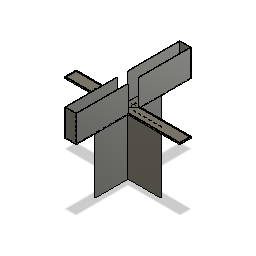
EPM (Autodesk Fusion 360 design; units mm, degrees)
Autodesk Fusion 360 part; units mm, degrees
note: some values were not read from the file. Chosen so that the rebuilt part matches the saved one: which bodies a step acts on. Set by a fixed rule: which sketch regions a step uses.
sketch "Maze" plane through (0, 0, 0) normal (0, 1, 0) x (1, 0, 0) in component "Main"
  line L0 (-50, 50) -> (50, 50) construction
  line L1 (50, 50) -> (50, -50) construction
  line L2 (50, -50) -> (-50, -50)
  line L3 (-50, -50) -> (-50, 50) construction
  line L4 (-50, 50) -> (-50, 550)
  line L5 (-50, 550) -> (50, 550)
  line L6 (50, 550) -> (50, 50)
  line L7 (50, 50) -> (550, 50)
  line L8 (550, 50) -> (550, -50)
  line L9 (550, -50) -> (50, -50)
  line L10 (-50, 50) -> (50, -50)
  line L11 (55.8, 55.8) -> (555.8, 55.8)
  line L12 (555.8, 55.8) -> (555.8, -55.8)
  line L13 (555.8, -55.8) -> (55.8, -55.8)
  line L14 (-50, -50) -> (-50, -550)
  line L15 (-50, -550) -> (50, -550)
  line L16 (50, -550) -> (50, -50)
  line L17 (55.8, -55.8) -> (55.8, -555.8)
  line L18 (55.8, -555.8) -> (-55.8, -555.8)
  line L19 (-50, 50) -> (-550, 50)
  line L20 (-550, 50) -> (-550, -50)
  line L21 (-550, -50) -> (-50, -50)
  line L22 (55.8, 55.8) -> (55.8, 555.8)
  line L23 (55.8, 555.8) -> (-55.8, 555.8)
  line L24 (-55.8, 555.8) -> (-55.8, 55.8)
  line L25 (-55.8, 55.8) -> (-555.8, 55.8)
  line L26 (-555.8, 55.8) -> (-555.8, -55.8)
  line L27 (-555.8, -55.8) -> (-55.8, -55.8)
  line L28 (-55.8, -55.8) -> (-55.8, -555.8)
  line L29 (-55.8, 55.8) -> (-50, 55.8)
  line L30 (-55.8, 55.8) -> (-55.8, 50)
  line L31 (55.8, 55.8) -> (50, 55.8)
  line L32 (55.8, 55.8) -> (55.8, 50)
  line L33 (-55.8, -55.8) -> (-55.8, -50)
  line L34 (-55.8, -55.8) -> (-50, -55.8)
  line L35 (55.8, -55.8) -> (55.8, -50)
  line L36 (55.8, -55.8) -> (50, -55.8)
  line L37 (-50, 550) -> (-50, 555.8)
  line L38 (550, 50) -> (555.8, 50)
  line L39 (50, -550) -> (50, -555.8)
  line L40 (-550, -50) -> (-555.8, -50)
  line L41 (-50, -50) -> (50, 50)
  line L42 (550, 50) -> (550, 55.8)
  line L43 (550, -50) -> (555.8, -50)
  line L44 (555.8, -50) -> (550, -50)
  line L45 (550, -50) -> (550, -55.8)
  line L46 (50, -550) -> (55.8, -550)
  line L47 (-50, -550) -> (-50, -555.8)
  line L48 (-50, -550) -> (-55.8, -550)
  line L49 (-550, -50) -> (-550, -55.8)
  line L50 (-550, 50) -> (-550, 55.8)
  line L51 (-550, 55.8) -> (-550, 50)
  line L52 (-555.8, 50) -> (-550, 50)
  line L53 (-50, 550) -> (-55.8, 550)
  line L54 (50, 550) -> (55.8, 550)
  line L55 (50, 550) -> (50, 555.8)
  line L56 (-55.8, 75.8) -> (-50, 75.8)
  line L57 (50, 75.8) -> (55.8, 75.8)
  line L58 (75.8, 55.8) -> (75.8, 50)
  line L59 (75.8, -50) -> (75.8, -55.8)
  line L60 (-50, 75.8) -> (50, 75.8) construction
  line L61 (75.8, 50) -> (75.8, -50) construction
  line L62 (-52.9, 75.8) -> (-52.9, 55.8) construction
  line L63 (75.8, 52.9) -> (55.8, 52.9) construction
  line L64 (-30, 555.8) -> (-30, 550)
  line L65 (-30, 552.9) -> (-50, 552.9) construction
  line L66 (550, 30) -> (555.8, 30)
  line L67 (552.9, 30) -> (552.9, 50) construction
  line L68 (2.9, 2.9) -> (-2.9, 2.9)
  line L69 (-2.9, 2.9) -> (-2.9, -2.9)
  line L70 (-2.9, -2.9) -> (2.9, -2.9)
  line L71 (2.9, -2.9) -> (2.9, 2.9)
  dimension "d8" = 100
  dimension "d9" = 500
  dimension "d13" = 5.8
  dimension "d33" = 20
  dimension "d34" = 20
  dimension "d108" = 5.8
  constraint horizontal L0
  constraint vertical L1
  constraint horizontal L2
  constraint vertical L3
  constraint perpendicular L0 L4
  constraint perpendicular L4 L5
  constraint perpendicular L0 L6
  constraint perpendicular L1 L7
  constraint perpendicular L7 L8
  constraint perpendicular L1 L9
  constraint equal L2 L3
  constraint midpoint origin L10
  constraint parallel L7 L11
  constraint perpendicular L11 L12
  constraint perpendicular L12 L13
  constraint perpendicular L2 L14
  constraint perpendicular L14 L15
  constraint perpendicular L13 L16
  constraint perpendicular L13 L17
  constraint perpendicular L17 L18
  constraint perpendicular L4 L19
  constraint perpendicular L19 L20
  constraint perpendicular L14 L21
  constraint equal L4 L19
  constraint equal L9 L19
  constraint equal L9 L16
  constraint perpendicular L11 L22
  constraint perpendicular L6 L23
  constraint perpendicular L23 L24
  constraint perpendicular L24 L25
  constraint perpendicular L25 L26
  constraint perpendicular L24 L27
  constraint perpendicular L15 L28
  constraint coincident L4 L29.end
  constraint perpendicular L4 L29
  constraint coincident L19 L30.end
  constraint perpendicular L19 L30
  constraint coincident L6 L31.end
  constraint perpendicular L6 L31
  constraint coincident L7 L32.end
  constraint perpendicular L7 L32
  constraint coincident L21 L33.end
  constraint perpendicular L21 L33
  constraint coincident L14 L34.end
  constraint perpendicular L14 L34
  constraint coincident L9 L35.end
  constraint perpendicular L9 L35
  constraint coincident L16 L36.end
  constraint perpendicular L16 L36
  constraint coincident L23 L37.end
  constraint perpendicular L23 L37
  constraint coincident L12 L38.end
  constraint perpendicular L12 L38
  constraint coincident L18 L39.end
  constraint perpendicular L18 L39
  constraint coincident L26 L40.end
  constraint perpendicular L26 L40
  constraint equal L29 L30
  constraint equal L29 L31
  constraint equal L31 L32
  constraint equal L32 L35
  constraint equal L35 L36
  constraint equal L34 L36
  constraint equal L33 L34
  constraint equal L33 L37
  constraint equal L37 L38
  constraint equal L38 L39
  constraint equal L39 L40
  constraint coincident L11 L42.end
  constraint perpendicular L11 L42
  constraint coincident L12 L43.end
  constraint perpendicular L12 L43
  constraint coincident L13 L45.end
  constraint perpendicular L13 L45
  constraint coincident L17 L46.end
  constraint perpendicular L17 L46
  constraint coincident L18 L47.end
  constraint perpendicular L18 L47
  constraint coincident L28 L48.end
  constraint perpendicular L28 L48
  constraint coincident L27 L49.end
  constraint perpendicular L27 L49
  constraint coincident L25 L50.end
  constraint perpendicular L25 L50
  constraint coincident L26 L52.start
  constraint perpendicular L50 L52
  constraint coincident L24 L53.end
  constraint perpendicular L24 L53
  constraint coincident L22 L54.end
  constraint perpendicular L22 L54
  constraint coincident L23 L55.end
  constraint perpendicular L23 L55
  constraint coincident L24 L56.start
  constraint coincident L4 L56.end
  constraint perpendicular L4 L56
  constraint coincident L6 L57.start
  constraint coincident L22 L57.end
  constraint perpendicular L22 L57
  constraint coincident L11 L58.start
  constraint coincident L7 L58.end
  constraint perpendicular L7 L58
  constraint coincident L9 L59.start
  constraint coincident L13 L59.end
  constraint perpendicular L13 L59
  constraint perpendicular L6 L60
  constraint perpendicular L7 L61
  constraint midpoint L56 L62.start
  constraint midpoint L29 L62.end
  constraint midpoint L58 L63.start
  constraint midpoint L32 L63.end
  constraint equal L62 L63
  constraint coincident L23 L64.start
  constraint coincident L5 L64.end
  constraint perpendicular L5 L64
  constraint midpoint L64 L65.start
  constraint midpoint L37 L65.end
  constraint coincident L8 L66.start
  constraint coincident L12 L66.end
  constraint perpendicular L12 L66
  constraint midpoint L66 L67.start
  constraint midpoint L38 L67.end
  constraint equal L65 L67
  constraint horizontal L68
  constraint vertical L69
  constraint horizontal L70
  constraint vertical L71
  constraint coincident L41 L69.end
  constraint coincident L41 L68.start
  constraint coincident L10 L68.end
  measures "d8" distance of L4.end L5.end
  measures "d9" distance of L0.start L4.end
  measures "d13" distance of L4.end L37.end
  measures "d33" distance of L62.start L62.end
  measures "d34" distance of L65.start L65.end
  measures "d108" distance of L68.start L68.end
sketch "Base" plane through (0, 0, 0) normal (0, 0, 1) x (1, 0, 0) in component "Main"
  line L0 (325, -5.8) -> (325, -595.75)
  line L1 (325, -595.75) -> (-325, -595.75)
  line L2 (-325, -595.75) -> (-325, -5.8)
  line L3 (-300, -5.8) -> (-300, 0)
  line L4 (-300, 0) -> (-325, 0)
  line L5 (-325, 0) -> (-325, -5.8)
  line L6 (325, -5.8) -> (325, 0)
  line L7 (325, 0) -> (300, 0)
  line L8 (300, 0) -> (300, -5.8)
  line L9 (300, 0) -> (-300, 0) construction
  line L10 (-300, -5.8) -> (-325, -5.8)
  line L11 (300, -5.8) -> (325, -5.8)
  line L12 (300, -5.8) -> (-300, -5.8)
  line L13 (0, 0) -> (0, -5.8) construction
  dimension "d79" = 650
  dimension "d119" = 589.95
  dimension "d121" = 5.8
  dimension "d122" = 25
  constraint vertical L0
  constraint perpendicular L0 L1
  constraint perpendicular L1 L2
  constraint perpendicular L3 L4
  constraint perpendicular L6 L7
  constraint equal L3 L8
  constraint coincident L3.end L4.start
  constraint perpendicular L5 L9
  constraint midpoint L13.start L9
  constraint perpendicular L4 L5
  constraint coincident L2.end L5.end
  constraint perpendicular L6 L11
  constraint perpendicular L3 L12
  constraint coincident L13.start origin
  constraint perpendicular L12 L13
  constraint coincident L12 L13.end
  constraint perpendicular L5 L10
  constraint perpendicular L2 L10
  constraint perpendicular L0 L11
  constraint coincident L4.end L5.start
  constraint equal L4 L7
  measures "d79" distance of L0.end L1.end
  measures "d119" distance of L1.end L2.end
  measures "d121" distance of L13.start L13.end
  measures "d122" distance of L3.end L4.end
sketch "Support1" plane through (0, 0, 0) normal (0, 0, 1) x (1, 0, 0) in component "Main"
  line L0 (-55.8, -5.8) -> (55.8, -5.8)
  line L1 (55.8, -5.8) -> (2.9, -61.6)
  line L2 (2.9, -61.6) -> (-2.9, -61.6)
  line L3 (-2.9, -61.6) -> (-55.8, -5.8)
  line L4 (0, -61.6) -> (0, -5.8) construction
  line L5 (0, 0) -> (0, -5.8) construction
  dimension "d133" = 111.6
  dimension "d134" = 5.8
  dimension "d135" = 55.8
  dimension "d136" = 5.8
  constraint horizontal L0
  constraint parallel L0 L2
  constraint midpoint L2 L4.start
  constraint perpendicular L0 L4
  constraint midpoint L0 L4.end
  constraint coincident L5.start origin
  constraint vertical L5
  constraint coincident L4.end L5.end
  measures "d133" distance of L0.start L0.end
  measures "d134" distance of L1.end L2.end
  measures "d135" distance of L4.start L4.end
  measures "d136" distance of L5.start L4.end
sketch "Support2" plane through (0, 0, 0) normal (0, 1, 0) x (1, 0, 0) in component "Main"
  line L0 (2.9, 2.9) -> (55.8, 2.9)
  line L1 (55.8, 2.9) -> (55.8, 55.8)
  line L2 (55.8, 55.8) -> (2.9, 55.8)
  line L3 (2.9, 55.8) -> (2.9, 2.9)
  line L4 (0, 0) -> (2.9, 0) construction
  line L5 (2.9, 0) -> (2.9, 2.9) construction
  dimension "d141" = 52.9
  dimension "d142" = 2.9
  constraint horizontal L0
  constraint vertical L1
  constraint horizontal L2
  constraint vertical L3
  constraint equal L0 L1
  constraint coincident L4.start origin
  constraint horizontal L4
  constraint perpendicular L0 L5
  constraint equal L4 L5
  constraint coincident L0.start L3.end
  measures "d141" distance of L0.start L0.end
  measures "d142" distance of L4.start L4.end
extrude "Extrude12" add sketch "Base" along normal mid plane 5.8 contours L0 L1 L2 L10 L11 L12 makes body 1 in component "Main"
extrude "Extrude13" add sketch "Base" along normal mid plane 5.8 contours L6 L7 L8 L11 bodies 1 in component "Main"
pattern_linear "R-Pattern4" count 6 spacing 50 along (-1, 0, 0) of "Extrude13" in component "Main"
extrude "Extrude14" add sketch "Base" along normal mid plane 5.8 contours L3 L4 L5 L10 bodies 1 in component "Main"
pattern_linear "R-Pattern5" count 6 spacing 50 along (1, 0, 0) of "Extrude14" in component "Main"
fillet "Fillet1" radius 10 2 edges at (-325, -595.75, 0) (325, -595.75, 0) on bodies 1 in component "Main"
pattern_circular "C-Pattern4" count 2 over 90 about axis through (0, 1.75, 0) along (0, 1, 0) of bodies 1 makes body 2 in component "Main"
extrude "Extrude15" cut sketch "Maze" against normal blind 294.975 from surface at -5.8 contours L10 L41 L70 | L10 L41 L71 | L10 L41 L69 | L10 L41 L68 bodies 1 in component "Main"
combine "Combine4" operation cut target body 2 tool bodies 1 keep tools in component "Main"
extrude "Extrude1" add sketch "Maze" against normal blind 5.8 separate body contours L10 L41 L68 | L4 L5 L6 L10 L41 L68 | L6 L22 L31 L57 | L4 L24 L29 L56 | L6 L22 L54 L57 | L4 L24 L53 L56 | L22 L23 L54 L55 | L5 L23 L55 L64 | L5 L23 L37 L64 | L23 L24 L37 L53 makes body 3 in component "Main"
extrude "Extrude4" cut sketch "Maze" against normal blind 5.8 contours L6 L22 L31 L57 | L4 L24 L29 L56 bodies 3 in component "Main"
pattern_linear "R-Pattern1" count 13 spacing 40 along (0, 0, -1) of "Extrude4" in component "Main"
extrude "Extrude7" cut sketch "Maze" against normal blind 5.8 contours L5 L23 L37 L64 bodies 3 in component "Main"
pattern_linear "R-Pattern2" count 3 spacing 40 along (1, 0, 0) of "Extrude7" in component "Main"
combine "Combine5" operation cut target body 3 tool bodies 2 keep tools in component "Main"
extrude "Extrude16" add sketch "Maze" along normal blind 4.25 separate body contours L10 L41 L68 | L4 L5 L6 L10 L41 L68 makes body 4 in component "Main"
extrude "Extrude5" add sketch "Maze" along normal blind 254.25 and the other way blind 5.8 separate body contours L6 L22 L31 L57 | L4 L24 L29 L56 | L6 L22 L54 L57 | L4 L24 L53 L56 | L22 L23 L54 L55 | L23 L24 L37 L53 makes body 5 at (-55.8, 167.5667, -222.4667) makes body 6 at (55.8, 167.5667, -389.1333) in component "Main"
extrude "Extrude6" add sketch "Maze" along normal blind 254.25 and the other way blind 5.8 separate body contours L5 L23 L55 L64 | L5 L23 L37 L64 makes body 7 in component "Main"
extrude "Extrude8" add sketch "Maze" along normal blind 19.5577 contours L22 L23 L54 L55 | L23 L24 L37 L53 bodies 7 in component "Main"
pattern_linear "R-Pattern3" count 7 spacing 39.1154 along (0, 1, 0) of "Extrude8" in component "Main"
extrude "Extrude9" add sketch "Maze" against normal blind 5.8 contours L22 L23 L54 L55 | L23 L24 L37 L53 bodies 7 in component "Main"
combine "Combine3" operation cut target body 7 tool bodies 3 keep tools in component "Main"
combine "Combine1" operation cut target body 5 tool bodies 3 7 keep tools in component "Main"
combine "Combine2" operation cut target body 6 tool bodies 3 7 keep tools in component "Main"
extrude "Extrude17" add sketch "Support1" against normal blind 5.8 from surface at -325 separate body makes body 8 in component "Main"
extrude "Extrude18" add sketch "Support2" against normal blind 5.8 from surface at -5.8 separate body makes body 9 in component "Main"
pattern_circular "C-Pattern3" count 4 over 360 about axis through (0, 1.75, 0) along (0, 1, 0) of bodies 3 5 6 7 4 8 9 makes body 10 at (-513.8667, -5.8, 3.3333) makes body 11 at (3.3333, -5.8, 513.8667) makes body 12 at (513.8667, -5.8, -3.3333) makes body 13 at (-300.5333, 169.5, 55.8) makes body 14 at (55.8, 169.5, 300.5333) makes body 15 at (300.5333, 169.5, -55.8) makes body 16 at (-300.5333, 169.5, -50) makes body 17 at (-50, 169.5, 300.5333) makes body 18 at (300.5333, 169.5, 55.8) makes body 19 at (-550, 39.1154, 3.3333) makes body 20 at (3.3333, 39.1154, 550) makes body 21 at (550, 39.1154, -3.3333) makes body 22 at (-233.8667, 4.25, 10) makes body 23 at (10, 4.25, 233.8667) makes body 24 at (233.8667, 4.25, -10) makes body 25 at (-325, -24.4, -0.9667) makes body 26 at (-0.9667, -24.4, 325) makes body 27 at (325, -24.4, 0.9667) makes body 28 at (-38.1667, -11.6, -20.5333) makes body 29 at (-20.5333, -11.6, 38.1667) makes body 30 at (38.1667, -11.6, 20.5333) in component "Main"
extrude "Extrude10" cut sketch "Maze" along normal through all from surface at 9.25 contours L9 L13 L35 L59 | L21 L27 L33 L49 | L9 L13 L45 L59 | L20 L26 L40 L52 | L26 L27 L40 L49 | L8 L12 L43 L44 L66 | L12 L13 L43 L44 L45 | L19 L25 L30 L50 L51 | L25 L26 L50 L51 L52 | L8 L12 L38 L66 | L7 L11 L32 L58 | L11 L12 L38 L42 | L7 L11 L42 L58 bodies 13 15 16 18 19 21 in component "Main"
extrude "Extrude11" add sketch "Maze" along normal blind 254.25 and the other way blind 5.8 contours L9 L16 L35 L36 | L14 L21 L33 L34 | L6 L7 L31 L32 | L4 L19 L29 L30 bodies 5 6 14 17 in component "Main"
fillet "Fillet2" radius 10 4 edges at (-52.9, 254.25, -50) (52.9, 254.25, -50) (52.9, 254.25, 50) (-52.9, 254.25, 50) on bodies 5 6 14 17 in component "Main"
component "Main" placed x (1, 0, 0) y (0, 1, 0) z (0, 0, 1) at (0, 0, 0)
hidden bodies 4
equation "d8 = Width"
equation "d9 = Length"
equation "d13 = Thick"
equation "d14 = -Thick"
equation "Width = 100 mm"
equation "Length = 500 mm"
equation "Height = 250 mm"
equation "Thick = 5.8 mm"
equation "nTabsL = 25"
equation "tabL = Length / nTabsL"
equation "nTabsW = 5"
equation "tabW = Width / nTabsW"
equation "nTabsH = 13"
equation "tabH = ( Height + FloorThick ) / nTabsH"
equation "d33 = tabL"
equation "d34 = tabW"
equation "d35 = -Thick"
equation "d37 = ( nTabsL + 1 ) / 2"
equation "d39 = -2 * tabL"
equation "d41 = Height + FloorThick"
equation "d43 = Thick"
equation "Lip = 5 mm"
equation "FloorThick = 4.25 mm"
equation "d47 = Height + FloorThick"
equation "d49 = Thick"
equation "d51 = -Thick"
equation "d53 = ( nTabsW + 1 ) / 2"
equation "d55 = 2 * tabW"
equation "d57 = tabH"
equation "d59 = ( nTabsH + 1 ) / 2"
equation "d61 = ( -2 * tabH )"
equation "d63 = -Thick"
equation "d72 = Lip + FloorThick"
equation "d74 = Height + FloorThick"
equation "d76 = Thick"
equation "d79 = BaseWidth"
equation "Lift = 600 mm"
equation "BaseWidth = 650 mm"
equation "BaseHeight = Lift - Thick - FloorThick"
equation "nTabsBase = 11"
equation "BaseTabOffset = 50 mm"
equation "tabB = ( BaseWidth / 2 - BaseTabOffset ) / nTabsBase"
equation "d92 = Thick"
equation "d94 = Thick"
equation "d96 = ( nTabsBase + 1 ) / 2"
equation "d98 = 2 * tabB"
equation "d100 = Thick"
equation "d102 = ( nTabsBase + 1 ) / 2"
equation "d104 = 2 * tabB"
equation "d108 = Thick"
equation "d109 = -Thick"
equation "d110 = -BaseHeight / 2"
equation "Fillet = 10 mm"
equation "d114 = Fillet"
equation "d116 = Fillet"
equation "d117 = FloorThick"
equation "d119 = BaseHeight"
equation "d121 = Thick"
equation "d122 = tabB"
equation "d133 = Width + 2 * Thick"
equation "d134 = Thick"
equation "d135 = Width / 2 + Thick"
equation "d136 = Thick"
equation "d138 = -Thick"
equation "d141 = Width / 2 + Thick / 2"
equation "d142 = Thick / 2"
equation "d143 = -Thick"
equation "d144 = -Thick"
named bodies: "Arm", "SdeWall1", "SideWall2", "BackWall", "Arm (1)", "Arm (2)", "Arm (3)", "Wall1 (1)", "Wall1 (2)", "Wall1 (3)", "Wall2 (1)", "Wall2 (2)", "Wall2 (3)", "Wall3 (1)", "Wall3 (2)", "Wall3 (3)", "Base1", "Base2", "Floor", "Floor (1)", "Floor (2)", "Floor (3)", "Support1", "Support (1)", "Support (2)", "Support (3)", "Support2", "Support2 (1)", "Support2 (2)", "Support2 (3)"
